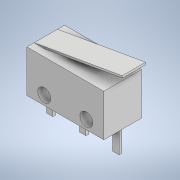
# Autodesk Inventor part: Endschalter
Saved by Autodesk Inventor 2021 (Build 250183000, 183)
## iProperties
Created: 2024-08-29
Part Number: Endschalter
Material: Generic
Document SubType Name: Modeling
Designer: Lukas
Density: 1 g/cm^3
Appearance: Default
Author: Lukas
Autodesk Inventor part; units mm, degrees
ref_plane "YZ Plane" through (0, 0, 0) normal (1, 0, 0) x (0, 1, 0)
ref_plane "XZ Plane" through (0, 0, 0) normal (0, 1, 0) x (-1, 0, 0)
ref_plane "XY Plane" through (0, 0, 0) normal (0, 0, 1) x (1, 0, 0)
sketch "Sketch1" plane through (0, 0, 0) normal (0, 0, 1) x (1, 0, 0)
  line L0 (-5.925, 3.25) -> (5.925, 3.25)
  line L1 (5.925, 3.25) -> (5.925, -3.25)
  line L2 (5.925, -3.25) -> (-5.925, -3.25)
  line L3 (-5.925, -3.25) -> (-5.925, 3.25)
  circle A0 centre (-3.25, -1.85) radius 1
  circle A1 centre (3.25, -1.85) radius 1
  point P0 (0, 0)
  point P1 (0, 3.25)
  point P2 (-5.925, 0)
  dimension "d0" = 11.85
  dimension "d1" = 6.5
  dimension "d2" = 1.4
  dimension "d3" = 6.5
  dimension "d4" = 3.25
  dimension "d5" = 2
  constraints: 8 end point, 2 centre point, 2 horizontal alignment, 2 midpoint, 2 parallel, 1 equal radius, 1 horizontal, 1 perpendicular, 1 vertical alignment
  measures "d0" distance of L0.start L0.end
  measures "d1" distance of L0.end L1.end
  measures "d2" distance from line of L2 A1.centre
  measures "d3" distance of A1.centre A0.centre
  measures "d4" horizontal distance of point (0, 0) A0.centre
  measures "d5" diameter of A0
extrude "Extrusion1" add sketch "Sketch1" along normal mid plane 5.8
sketch "Sketch2" plane through (0, 0, 0) normal (0, 0, 1) x (1, 0, 0)
  line L0 (-5.925, 3.25) -> (5.925, 3.25) projected
  line L1 (-5.925, 3.25) -> (7.6653, 5.6463)
  line L2 (7.6653, 5.6463) -> (7.7174, 5.3509)
  line L3 (7.7174, 5.3509) -> (-4.1974, 3.25)
  point P0 (0, 0)
  dimension "d9" = 0.3
  dimension "d10" = 10
  dimension "d11" = 13.8
  constraints: 6 end point, 1 parallel, 1 perpendicular, 1 point on line
  measures "d9" distance between parallel lines of L1 L3
  measures "d10" angle of L0 L3
  measures "d11" distance of L0.start L1.end
extrude "Extrusion2" add sketch "Sketch2" along normal mid plane 3.6
sketch "Sketch3" plane through (0, 0, 0) normal (0, 0, 1) x (1, 0, 0)
  line L0 (-5.925, -3.25) -> (5.925, -3.25) projected
  line L1 (-5.6, -3.25) -> (-4.6, -3.25)
  line L2 (-4.6, -3.25) -> (-4.6, -6.75)
  line L3 (-4.6, -6.75) -> (-5.6, -6.75)
  line L4 (-5.6, -6.75) -> (-5.6, -3.25)
  line L5 (-0.5, -3.25) -> (0.5, -3.25)
  line L6 (0.5, -3.25) -> (0.5, -6.75)
  line L7 (0.5, -6.75) -> (-0.5, -6.75)
  line L8 (-0.5, -6.75) -> (-0.5, -3.25)
  line L9 (4.6, -3.25) -> (5.6, -3.25)
  line L10 (5.6, -3.25) -> (5.6, -6.75)
  line L11 (5.6, -6.75) -> (4.6, -6.75)
  line L12 (4.6, -6.75) -> (4.6, -3.25)
  point P0 (0, 0)
  point P1 (0, -6.75)
  point P2 (0, -3.25)
  dimension "d14" = 3.5
  dimension "d15" = 10.2
  dimension "d16" = 5.1
  dimension "d17" = 1
  constraints: 24 end point, 6 parallel, 4 point on line, 3 horizontal, 3 perpendicular, 2 collinear, 2 midpoint, 1 horizontal alignment, 1 vertical alignment
  measures "d14" distance of L3.end L1.start
  measures "d15" distance between parallel lines of L10 L2
  measures "d16" distance between parallel lines of L6 L2
  measures "d17" distance of L2.end L3.end
extrude "Extrusion3" add sketch "Sketch3" along normal mid plane 0.45
equation "\"d4\" = 0.5 * d3"
equation "\"d16\" = 0.5 * d15"
body "Solid1"
